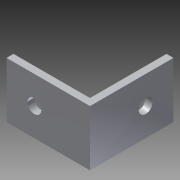
# Autodesk Inventor part: L-Bracket
Saved by Autodesk Inventor 2013 (Build 170138000, 138)
## iProperties
Created: 2013-07-19
Part Number: L-Bracket
Material: Aluminum 6061
Document SubType Name: Modeling
Designer: robotics
Density: 1 g/cm^3
Author: robotics
Autodesk Inventor part; units mm, degrees
ref_plane "YZ Plane" through (0, 0, 0) normal (1, 0, 0) x (0, 1, 0)
ref_plane "XZ Plane" through (0, 0, 0) normal (0, 1, 0) x (-1, 0, 0)
ref_plane "XY Plane" through (0, 0, 0) normal (0, 0, 1) x (1, 0, 0)
sketch "Sketch1" plane through (0, 0, 0) normal (0, 1, 0) x (-1, 0, 0)
  line L0 (0, 0) -> (-38.1, 0)
  line L1 (-38.1, 0) -> (-38.1, -38.1)
  line L2 (-38.1, -38.1) -> (-34.925, -38.1)
  line L3 (-34.925, -38.1) -> (-34.925, -3.175)
  line L4 (-34.925, -3.175) -> (0, -3.175)
  line L5 (0, -3.175) -> (0, 0)
  dimension "d0" = 38.1
  dimension "d1" = 38.1
  dimension "d2" = 3.175
  dimension "d3" = 3.175
  constraints: 12 end point, 4 parallel, 1 horizontal, 1 perpendicular
  measures "d0" distance of L0.start L0.end
  measures "d1" distance of L0.end L1.end
  measures "d2" distance of L4.end L0.start
  measures "d3" distance between parallel lines of L3 L1
extrude "Extrusion1" add sketch "Sketch1" along normal blind 25.4
sketch "Sketch2" plane through (38.1, 0, 0) normal (1, 0, 0) x (0, 0, -1)
  line L0 (0, 0) -> (38.1, 0) projected
  line L1 (38.1, 0) -> (38.1, 25.4) projected
  line L2 (0, 25.4) -> (38.1, 25.4) projected
  line L3 (0, 0) -> (0, 25.4) projected
sketch "Sketch3" plane through (0, 0, 0) normal (0, 0, 1) x (1, 0, 0)
  line L0 (0, 25.4) -> (38.1, 25.4) projected
  line L1 (0, 0) -> (0, 25.4) projected
  point P0 (12.7, 12.7)
  dimension "d6" = 12.7
  dimension "d7" = 12.7
  measures "d6" distance from line of L1 point (12.7, 12.7)
  measures "d7" distance from line of point (12.7, 12.7) L0
hole "Hole1" at (12.7, 12.7, 0) direction (0, 0, -1) diameter 6.35 end through all
sketch "Sketch4" plane through (38.1, 0, 0) normal (1, 0, 0) x (0, 0, -1)
  line L0 (0, 0) -> (38.1, 0) projected
  line L1 (38.1, 0) -> (38.1, 25.4) projected
  line L2 (0, 0) -> (0, 25.4) projected
  point P0 (25.4, 12.7)
  dimension "d15" = 12.7
  dimension "d16" = 12.7
  dimension "d24" = 25.4
  measures "d15" distance from line of point (25.4, 12.7) L1
  measures "d16" distance from line of L0 point (25.4, 12.7)
  measures "d24" distance from line of L2 point (25.4, 12.7)
hole "Hole2" at (38.1, 12.7, -25.4) direction (-1, 0, 0) diameter 6.35 end through all
body "Solid1"
